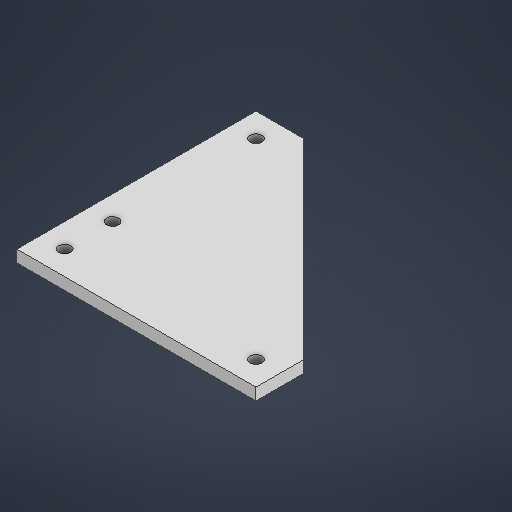
# Autodesk Inventor part: soporte tipo triangulo
Saved by Autodesk Inventor 2026.1 (Build 301233020, 233B)
## iProperties
Created: 2025-11-01
Part Number: soporte tipo triangulo
Material: Generic
Document SubType Name: Modeling
Designer: Tito Luyo Murata
Density: 1 g/cm^3
Appearance: Default
Author: Tito Luyo Murata
Autodesk Inventor part; units mm, degrees
ref_plane "YZ Plane" through (0, 0, 0) normal (1, 0, 0) x (0, 1, 0)
ref_plane "XZ Plane" through (0, 0, 0) normal (0, 1, 0) x (-1, 0, 0)
ref_plane "XY Plane" through (0, 0, 0) normal (0, 0, 1) x (1, 0, 0)
sketch "Sketch1" plane through (0, 0, 0) normal (0, 1, 0) x (-1, 0, 0)
  line L0 (0, 0) -> (0, -100)
  line L1 (0, -100) -> (-20, -100)
  line L2 (0, 0) -> (-100, 0)
  line L3 (-100, 0) -> (-100, -20)
  line L4 (-100, -20) -> (-20, -100)
  line L5 (26.0864, -10) -> (-132.7995, -10) construction
  line L6 (-10, 33.7229) -> (-10, -136.0235) construction
  circle A0 centre (-10, -10) radius 2.5
  circle A1 centre (-10, -90) radius 2.5
  circle A2 centre (-10, -30) radius 2.5
  circle A3 centre (-90, -10) radius 2.5
  dimension "d0" = 100
  dimension "d1" = 20
  dimension "d2" = 100
  dimension "d3" = 20
  dimension "d4" = 10
  dimension "d5" = 10
  dimension "d6" = 5
  dimension "d7" = 5
  dimension "d8" = 5
  dimension "d9" = 5
  dimension "d10" = 10
  dimension "d11" = 30
  dimension "d12" = 10
  constraints: 14 end point, 5 point on line, 4 centre point, 2 horizontal, 2 perpendicular, 2 vertical
  measures "d0" distance of L0.start L0.end
  measures "d1" distance of L0.end L1.end
  measures "d2" distance of L0.start L2.end
  measures "d3" distance of L2.end L3.end
  measures "d4" distance between parallel lines of L2 L5
  measures "d5" distance between parallel lines of L0 L6
  measures "d6" diameter of A0
  measures "d7" diameter of A1
  measures "d8" diameter of A2
  measures "d9" diameter of A3
  measures "d10" distance from line of L1 A1.centre
  measures "d11" distance from line of L2 A2.centre
  measures "d12" distance from line of L3 A3.centre
extrude "Extrusion1" add sketch "Sketch1" along normal blind 5
equation "\"d0\" = dimension"
equation "\"d1\" = perfil_ancho"
equation "\"d2\" = dimension"
equation "\"d3\" = perfil_ancho"
equation "\"d4\" = 0.5 * perfil_ancho"
equation "\"d5\" = 0.5 * perfil_ancho"
equation "\"d6\" = hueco_diametro"
equation "\"d7\" = hueco_diametro"
equation "\"d8\" = hueco_diametro"
equation "\"d9\" = hueco_diametro"
equation "\"d10\" = separación"
equation "\"d11\" = perfil_ancho + separación"
equation "\"d12\" = separación"
equation "\"d13\" = espesor"
equation "\"perfil_ancho\" = 20"
equation "\"hueco_diametro\" = 5"
equation "\"dimension\" = 100"
equation "\"separación\" = 10"
equation "\"espesor\" = 5"
body "Solid1"
